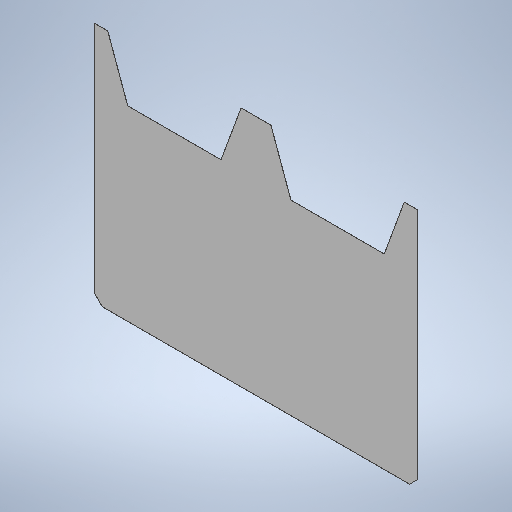
# Autodesk Inventor part: GBK-RK-0015 partition 5
Saved by Autodesk Inventor 2026 (Build 300175000, 175)
## iProperties
Created: 2026-09-14
Part Number: GBK-RK-0015 partition 5
Material: Generic
Document SubType Name: Sheet Metal
Designer: admin
Density: 1 g/cm^3
Sheet Metal Rule: По умолчанию_мм
Appearance: Default
Author: admin
Autodesk Inventor part; units mm, degrees
ref_plane "YZ Plane" through (0, 0, 0) normal (1, 0, 0) x (0, 1, 0)
ref_plane "XZ Plane" through (0, 0, 0) normal (0, 1, 0) x (-1, 0, 0)
ref_plane "XY Plane" through (0, 0, 0) normal (0, 0, 1) x (1, 0, 0)
sketch "Sketch3" plane through (0, 0, 0) normal (0, 0, 1) x (1, 0, 0)
  line L0 (735, 1100) -> (735, 35.3553)
  line L1 (735, 35.3553) -> (699.6447, 0)
  line L2 (699.6447, 0) -> (-699.6447, 0)
  line L3 (-699.6447, 0) -> (-735, 35.3553)
  line L4 (-735, 35.3553) -> (-735, 1100)
  line L5 (-735, 1100) -> (735, 1100)
  line L6 (0, 0) -> (0, 1100) construction
  line L7 (675, 1100) -> (584.0074, 850)
  line L8 (584.0074, 850) -> (159.0074, 850)
  line L9 (159.0074, 850) -> (68.0149, 1100)
  line L10 (-68.0149, 1100) -> (-159.0074, 850)
  line L11 (-159.0074, 850) -> (-584.0074, 850)
  line L12 (-584.0074, 850) -> (-675, 1100)
  dimension "d25" = 50
  dimension "d26" = 1100
  dimension "d27" = 1470
  dimension "d32" = 425
  dimension "d33" = 60
  dimension "d35" = 250
  dimension "d38" = 110
  measures "d25" distance of L2.end L3.end
  measures "d26" distance between parallel lines of L2 L5
  measures "d27" distance of L4.end L0.start
  measures "d32" distance of L10.end L11.end
  measures "d33" distance of L12.end L4.end
  measures "d35" distance between parallel lines of L11 L5
  measures "d38" angle of L11 L12
extrude "Plate3" add sketch "Sketch3" along normal blind 0.5 contours L0 L1 L2 L3 L4 L5 L12 L11 L10 L9 L8 L7
equation "\"d28\" = Thickness"
equation "\"BendRadius\" = Thickness"
equation "\"BendReliefWidth\" = Thickness"
equation "\"BendReliefDepth\" = 0.5 * Thickness"
equation "\"CornerReliefSize\" = 4 * Thickness"
equation "\"MinimumRemnant\" = 2 * Thickness"
equation "\"TransitionRadius\" = BendRadius"
equation "\"JacobiRadiusSize\" = BendRadius"
equation "\"GapSize\" = Thickness"
equation "\"Thickness\" = 0.5"
body "Solid2"
